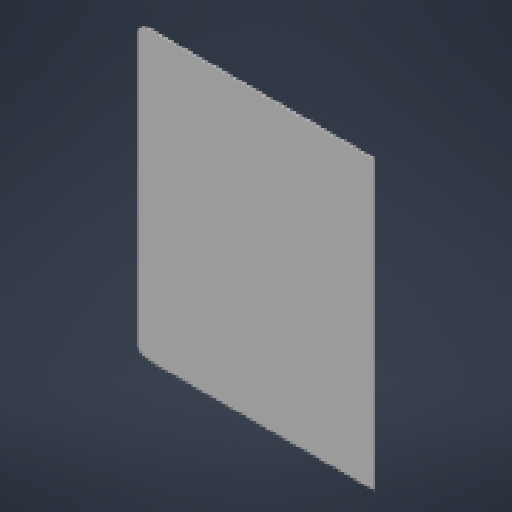
# Autodesk Inventor part: Top Cover
Saved by Autodesk Inventor 2023 (Build 270158000, 158)
## iProperties
Created: 2022-10-09
Part Number: Top Cover
Material: Aluminum 6061
Document SubType Name: Modeling
Designer: Hilal Yahya
Density: 2.7 g/cm^3
Appearance: Aluminum - Flat
Author: Hilal Yahya
Autodesk Inventor part; units mm, degrees
ref_plane "YZ Plane" through (0, 0, 0) normal (1, 0, 0) x (0, 1, 0)
ref_plane "XZ Plane" through (0, 0, 0) normal (0, 1, 0) x (-1, 0, 0)
ref_plane "XY Plane" through (0, 0, 0) normal (0, 0, 1) x (1, 0, 0)
sketch "Sketch1" plane through (0, 0, 0) normal (0, 0, 1) x (1, 0, 0)
  line L0 (-167.701, 0) -> (65.3284, 0) projected
  line L1 (76.0929, 0) -> (65.3284, 0) projected
  ellipse E0 centre (76.0929, 10) end of major axis (76.0929, 20) minor radius 7.0711 (76.0929, 0) -> (83.164, 10) ccw projected
  line L2 (83.164, 290) -> (83.164, 10) projected
  ellipse E1 centre (76.0929, 290) end of major axis (76.0929, 280) minor radius 7.0711 (83.164, 290) -> (76.0929, 300) ccw projected
  line L3 (65.3284, 300) -> (76.0929, 300) projected
  line L4 (65.3284, 300) -> (-167.701, 300) projected
  line L5 (-181.8431, 290) -> (-181.8431, 10) projected
  ellipse E2 centre (-167.701, 10) end of major axis (-181.8431, 10) minor radius 10 (-181.8431, 10) -> (-167.701, 0) ccw projected
  ellipse E3 centre (-167.701, 290) end of major axis (-153.5589, 290) minor radius 10 (-167.701, 300) -> (-181.8431, 290) ccw projected
  line L6 (65.3284, 300) -> (65.3284, 0)
  point P0 (0, 0)
  constraints: 2 end point, 1 perpendicular, 4 other
extrude "Extrusion1" add sketch "Sketch1" against normal blind 1 contours E2 L5 E3 L4 L6 L0
ref_plane "Work Plane1" through (-51.1863, 0, 116.5147) normal (-0.7071, 0, -0.7071) x (-0.7071, 0, 0.7071)
sketch "Sketch2" plane through (-51.1863, 0, 116.5147) normal (-0.7071, 0, -0.7071) x (-0.7071, 0, 0.7071)
  line L0 (-164.7767, 0) -> (-164.7767, 300) projected
  line L1 (-190, 290) -> (-190, 10) projected
  arc A0 (-190, 10) -> (-180, 0) centre (-180, 10) ccw projected
  line L2 (-180, 0) -> (-164.7767, 0) projected
  line L3 (-164.7767, 300) -> (-180, 300) projected
  arc A1 (-180, 300) -> (-190, 290) centre (-180, 290) ccw projected
  point P0 (-118.5825, 0)
extrude "Extrusion2" add sketch "Sketch2" along normal blind 1
body "Solid1"
